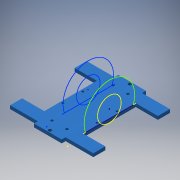
# Autodesk Inventor part: Base
Saved by Autodesk Inventor 2016 (Build 200138000, 138)
## iProperties
Created: 2017-02-20
Part Number: Base
Material: Generic
Document SubType Name: Modeling
Designer: jorge
Density: 1 g/cm^3
Appearance: Cyan
Author: jorge
Autodesk Inventor part; units mm, degrees
ref_plane "YZ Plane" through (0, 0, 0) normal (1, 0, 0) x (0, 1, 0)
ref_plane "XZ Plane" through (0, 0, 0) normal (0, 1, 0) x (-1, 0, 0)
ref_plane "XY Plane" through (0, 0, 0) normal (0, 0, 1) x (1, 0, 0)
sketch "Sketch1" plane through (0, 0, 0) normal (0, 1, 0) x (-1, 0, 0)
  line L0 (25, 0) -> (50, 0)
  line L1 (50, -75) -> (25, -75)
  line L2 (75, 0) -> (75, -25)
  line L3 (75, -25) -> (72, -25)
  line L4 (75, -75) -> (75, -50)
  line L5 (75, -50) -> (72, -50)
  line L6 (72, -50) -> (72, -25)
  line L7 (0, -25) -> (3, -25)
  line L8 (3, -25) -> (3, -50)
  line L9 (3, -50) -> (0, -50)
  line L10 (0, -75) -> (3, -75)
  line L11 (25, -75) -> (25, -72)
  line L12 (25, -72) -> (0, -72)
  line L13 (75, -75) -> (72, -75)
  line L14 (50, -75) -> (50, -72)
  line L15 (50, -72) -> (75, -72)
  line L16 (50, 0) -> (50, -3)
  line L17 (50, -3) -> (75, -3)
  line L18 (25, 0) -> (25, -3)
  line L19 (25, -3) -> (0, -3)
  line L20 (75, 0) -> (75, -25)
  line L21 (75, -50) -> (75, -75)
  line L22 (0, -75) -> (0, -50)
  line L23 (0, -25) -> (0, 0)
  dimension "d0" = 75
  dimension "d1" = 75
  dimension "d2" = 25
  dimension "d3" = 3
  dimension "d4" = 25
  dimension "d5" = 3
  dimension "d6" = 25
  dimension "d7" = 3
  dimension "d8" = 25
  dimension "d9" = 3
  dimension "d10" = 3
  constraints: 48 end point, 11 perpendicular, 10 point on line, 7 parallel, 2 horizontal, 1 vertical
  measures "d0" distance of L4.start L10.start
  measures "d1" distance of L2.start L4.start
  measures "d2" distance of L2.start L2.end
  measures "d3" distance of L2.end L3.end
  measures "d4" distance of L4.start L4.end
  measures "d5" distance of L7.start L7.end
  measures "d6" distance of L1.end L10.start
  measures "d7" distance of L1.end L11.end
  measures "d8" distance of L1.start L4.start
  measures "d9" distance of L0.end L16.end
  measures "d10" distance of L0.start L18.end
extrude "Extrusion1" add sketch "Sketch1" along normal blind 3
sketch "Sketch3" plane through (0, 0, 0) normal (0, -1, 0) x (1, 0, 0)
  line L0 (-3, -13.8146) -> (0, -13.8146) projected
  line L1 (0, -61.1854) -> (-3, -61.1854) projected
  line L2 (-72, -61.1854) -> (-75, -61.1854) projected
  line L3 (-75, -13.8146) -> (-72, -13.8146) projected
  line L4 (0, -61.1854) -> (-20, -61.1854)
  line L5 (-20, -61.1854) -> (-20, -13.8146)
  line L6 (0, -13.8146) -> (-20, -13.8146)
  line L7 (-75, -13.8146) -> (-55, -13.8146)
  line L8 (-55, -13.8146) -> (-55, -61.1854)
  line L9 (-75, -61.1854) -> (-55, -61.1854)
  line L10 (-75, -61.1854) -> (-75, -13.8146)
  line L11 (0, -13.8146) -> (0, -61.1854)
  line L12 (0, -50) -> (0, -72) projected
  point P0 (0, 0)
  dimension "d13" = 20
  dimension "d14" = 20
  constraints: 16 end point, 5 perpendicular, 2 point on line, 1 collinear, 1 horizontal
  measures "d13" distance of L1.start L4.end
  measures "d14" distance of L3.start L7.end
extrude "Extrusion2" cut sketch "Sketch3" along normal mid plane 25.4
sketch "Sketch4" plane through (0, 0, 0) normal (0, -1, 0) x (1, 0, 0)
  circle A0 centre (-30.7671, -9.9986) radius 1.14 projected
  circle A1 centre (-44.2271, -10.0014) radius 1.14 projected
  arc A2 (-31.5, -28.5) -> (-33.5, -28.5) centre (-32.5, -28.5) ccw projected
  circle A3 centre (-30.7671, -64.9995) radius 1.14 projected
  circle A4 centre (-44.2271, -65.0005) radius 1.14 projected
  arc A5 (-41.5, -28.5) -> (-43.5, -28.5) centre (-42.5, -28.5) ccw projected
  circle A6 centre (-42.5, -28.5) radius 1
  circle A7 centre (-32.5, -28.5) radius 1
  circle A8 centre (-30.7671, -64.9995) radius 1.14
  circle A9 centre (-44.2271, -65.0005) radius 1.14
  circle A10 centre (-44.2271, -10.0014) radius 1.14
  circle A11 centre (-30.7671, -9.9986) radius 1.14
  arc A12 (-33.5, -46.5) -> (-31.5, -46.5) centre (-32.5, -46.5) ccw projected
  arc A13 (-43.5, -46.5) -> (-41.5, -46.5) centre (-42.5, -46.5) ccw projected
  circle A14 centre (-32.5, -46.5) radius 1
  circle A15 centre (-42.5, -46.5) radius 1
  point P0 (0, 0)
  constraints: 8 coincident, 6 centre point, 4 concentric, 2 horizontal alignment, 4 other
extrude "Extrusion3" cut sketch "Sketch4" against normal blind 3 contours A0 | A1 | A3 | A4
sketch "Sketch5" plane through (0, 0, 0) normal (0, -1, 0) x (1, 0, 0)
  line L0 (-17.5, -6) -> (-17.5, -17) projected
  line L1 (-17.5, -17) -> (-29.5, -17) projected
  line L2 (-47, -17) -> (-56, -17) projected
  line L3 (-56, -6) -> (-56, -17) projected
  line L4 (-17.5, -17) -> (-29.5, -17)
  line L5 (-29.5, -17) -> (-29.5, -6)
  line L6 (-29.5, -6) -> (-17.5, -6)
  line L7 (-17.5, -6) -> (-17.5, -17)
  line L8 (-56, -17) -> (-47, -17)
  line L9 (-47, -17) -> (-47, -6)
  line L10 (-47, -6) -> (-56, -6)
  line L11 (-56, -6) -> (-56, -17)
  arc A0 (-23.098, -46.5011) -> (-21.098, -46.5011) centre (-22.098, -46.5011) ccw projected
  circle A1 centre (-22.098, -28.5012) radius 1 projected
  arc A2 (-21.098, -28.5011) -> (-23.098, -28.5011) centre (-22.098, -28.5011) ccw projected
  arc A3 (-23.098, -46.5011) -> (-21.098, -46.5011) centre (-22.098, -46.5011) ccw projected
  circle A4 centre (-22.098, -46.5078) radius 1 projected
  line L12 (-72, -25) -> (-72, -3) projected
  line L13 (-25, -3) -> (-3, -3) projected
  line L14 (-50, -72) -> (-72, -72) projected
  circle A5 centre (-52.902, -46.4986) radius 1 projected
  arc A6 (-51.902, -28.4986) -> (-53.902, -28.4986) centre (-52.902, -28.4986) ccw projected
  circle A7 centre (-52.902, -28.492) radius 1 projected
  circle A8 centre (-37.5, -1.5) radius 1.5 projected
  circle A9 centre (-1.5, -37.5) radius 1.5 projected
  circle A10 centre (-37.5, -73.5) radius 1.5 projected
  circle A11 centre (-73.5, -36) radius 1.5 projected
  circle A12 centre (-73.5, -36) radius 1.5 projected
  circle A13 centre (-73.5, -36) radius 1.5 projected
  circle A14 centre (-37.5, -1.5) radius 1.5 projected
  circle A15 centre (-37.5, -73.5) radius 1.5 projected
  circle A16 centre (-37.5, -73.5) radius 1.5 projected
  line L15 (-72, -50) -> (-75, -50) projected
  circle A17 centre (-37.5, -73.5) radius 1.5 projected
  circle A18 centre (-37.5, -73.5) radius 1.5 projected
  circle A19 centre (-37.5, -73.5) radius 1.5 projected
  circle A20 centre (-37.5, -73.5) radius 1.5 projected
  circle A21 centre (-37.5, -73.5) radius 1.5 projected
  circle A22 centre (-37.5, -73.5) radius 1.5 projected
  circle A23 centre (-37.5, -73.5) radius 1.5 projected
  circle A24 centre (-37.5, -73.5) radius 1.5 projected
  circle A25 centre (-37.5, -73.5) radius 1.5 projected
  circle A26 centre (-37.5, -73.5) radius 1.5 projected
  circle A27 centre (-37.5, -73.5) radius 1.5 projected
  circle A28 centre (-37.5, -73.5) radius 1.5 projected
  circle A29 centre (-37.5, -1.5) radius 1.5 projected
  circle A30 centre (-37.5, -73.5) radius 1.5 projected
  circle A31 centre (-37.5, -73.5) radius 1.5 projected
  circle A32 centre (-36.0014, -62.75) radius 1.5 projected
  line L16 (-50, -72) -> (-50, -75.5) projected
  line L17 (-72, -72) -> (-72, -50) projected
  line L18 (-75, -50) -> (-75, -25) projected
  line L19 (-75, -25) -> (-72, -25) projected
  line L20 (-72, -3) -> (-50, -3) projected
  line L21 (-50, -3) -> (-50, 0.5) projected
  line L22 (-25, 0.5) -> (-50, 0.5) projected
  line L23 (-25, -3) -> (-25, 0.5) projected
  line L24 (-3, -3) -> (-3, -25) projected
  line L25 (-3, -25) -> (0, -25) projected
  line L26 (0, -25) -> (0, -50) projected
  line L27 (0, -50) -> (-3, -50) projected
  line L28 (-3, -50) -> (-3, -72) projected
  line L29 (-3, -72) -> (-25, -72) projected
  line L30 (-25, -72) -> (-25, -75.5) projected
  line L31 (-50, -75.5) -> (-25, -75.5) projected
  point P0 (0, 0)
  point P1 (-37.5, -1.5)
  point P2 (-37.5, 0)
  constraints: 16 end point, 4 parallel, 2 horizontal, 2 perpendicular, 1 vertical alignment
extrude "Extrusion4" cut sketch "Sketch5" against normal blind 25.4 contours A4 A0 | A0 A4 | A1 | A5 | A7 A6 | A6 A7
sketch "Sketch6" plane through (0, 0, 0) normal (0, -1, 0) x (1, 0, 0)
  circle A0 centre (-52.902, -46.4986) radius 1 projected
  arc A1 (-21.098, -28.5011) -> (-23.098, -28.5011) centre (-22.098, -28.5011) ccw projected
  arc A2 (-23.098, -28.5011) -> (-21.098, -28.5011) centre (-22.098, -28.5012) ccw projected
  circle A3 centre (-22.098, -46.5078) radius 1 projected
  circle A4 centre (-52.902, -28.492) radius 1 projected
  circle A5 centre (-30.7671, -64.9995) radius 1.14 projected
  circle A6 centre (-30.7671, -9.9986) radius 1.14 projected
  circle A7 centre (-44.2271, -10.0014) radius 1.14 projected
  circle A8 centre (-44.2271, -65.0005) radius 1.14 projected
  line L0 (0, -61.1854) -> (-20, -61.1854) projected
  line L1 (-20, -61.1854) -> (-20, -13.8146) projected
  line L2 (-20, -13.8146) -> (0, -13.8146) projected
  line L3 (0, -3) -> (0, -13.8146) projected
  line L4 (-25, -3) -> (0, -3) projected
  line L5 (-25, 0) -> (-25, -3) projected
  line L6 (-50, 0) -> (-25, 0) projected
  line L7 (-50, -3) -> (-50, 0) projected
  line L8 (-75, -3) -> (-50, -3) projected
  line L9 (-75, -13.8146) -> (-75, -3) projected
  line L10 (-75, -13.8146) -> (-55, -13.8146) projected
  line L11 (-55, -13.8146) -> (-55, -61.1854) projected
  line L12 (-55, -61.1854) -> (-75, -61.1854) projected
  line L13 (-75, -72) -> (-75, -61.1854) projected
  line L14 (-50, -72) -> (-75, -72) projected
  line L15 (-50, -75) -> (-50, -72) projected
  line L16 (-25, -75) -> (-50, -75) projected
  line L17 (-25, -72) -> (-25, -75) projected
  line L18 (0, -72) -> (-25, -72) projected
  line L19 (0, -61.1854) -> (0, -72) projected
  circle A9 centre (-37.5, -73.5) radius 1.5
  circle A10 centre (-37.5, -1.5) radius 1.5
  point P0 (0, 0)
  dimension "d21" = 3
  dimension "d25" = 3
  constraints: 2 centre point
  measures "d21" diameter of A9
  measures "d25" diameter of A10
extrude "Extrusion5" cut sketch "Sketch6" against normal blind 25.4 contours A10 | A9
sketch "Sketch7" plane through (-50, 0, 0) normal (0, 0, 1) x (1, 0, 0)
  line L0 (12.5, 0) -> (12.5, 3) projected
  line L1 (12.5, 0) -> (25, 0) projected
  line L2 (25, 0) -> (25, 3) projected
  line L3 (12.5, 3) -> (25, 3) projected
  line L4 (0, 3) -> (12.5, 3) projected
  line L5 (0, 0) -> (0, 3) projected
  line L6 (0, 0) -> (12.5, 0) projected
  line L7 (12.5, 0) -> (12.5, 3) projected
  line L8 (0, 3) -> (12.5, 3) projected
  line L9 (0, 0) -> (0, 3) projected
  line L10 (0, 0) -> (12.5, 0) projected
  line L11 (12.5, 0) -> (25, 0) projected
  line L12 (25, 0) -> (25, 3) projected
  line L13 (12.5, 3) -> (25, 3) projected
  point P0 (50, 0)
extrude "Extrusion6" add sketch "Sketch7" along normal blind 0.5
sketch "Sketch8" plane through (-50, 0, -75) normal (0, 0, -1) x (-1, 0, 0)
  line L0 (0, 0) -> (-25, 0) projected
  line L1 (-25, 0) -> (-25, 3) projected
  line L2 (-25, 3) -> (0, 3) projected
  line L3 (0, 3) -> (0, 0) projected
  point P0 (-50, 0)
extrude "Extrusion7" add sketch "Sketch8" along normal blind 0.5
body "Solid1"
